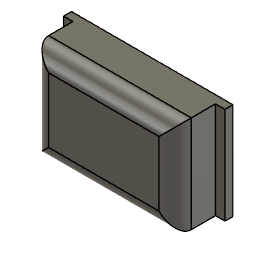
Side-Button (Autodesk Fusion 360 design; units mm, degrees)
Autodesk Fusion 360 part; units mm, degrees
sketch "Sketch1" plane through (0, 0, 0) normal (0, 0, 1) x (1, 0, 0)
  line L0 (-30, 20) -> (-12.335, 20)
  line L1 (-12.335, 20) -> (-12.335, 8)
  line L2 (-12.335, 8) -> (-30, 8)
  line L3 (-30, 8) -> (-30, 20)
  dimension "d1" = 17.665
  dimension "d2" = 12
  constraint horizontal L0
  constraint vertical L1
  constraint horizontal L2
  constraint vertical L3
  measures "d1" distance of L0.start L0.end
  measures "d2" distance of L0.start L2.end
extrude "Extrude1" add sketch "Sketch1" along normal blind 6
fillet "Fillet1" radius 2 4 edges at (-21.1675, 20, 6) (-12.335, 14, 6) (-30, 14, 6) (-21.1675, 8, 6)
sketch "Sketch2" plane through (0, 0, 0) normal (0, 0, -1) x (-1, 0, 0)
  line L0 (12.335, 8) -> (30, 8)
  line L1 (30, 8) -> (30, 20)
  line L2 (30, 20) -> (12.335, 20)
  line L3 (12.335, 20) -> (12.335, 8)
  line L4 (11.1675, 20) -> (31.1675, 20)
  line L5 (11.1675, 8) -> (31.1675, 8)
  line L6 (31.1675, 20) -> (31.1675, 8)
  line L7 (11.1675, 8) -> (11.1675, 20)
  point P0 (21.1675, 20)
  point P1 (21.1675, 8)
  dimension "d7" = 20
  constraint midpoint L4 P0
  constraint coincident L2 P0
  constraint parallel L2 L4
  constraint midpoint L5 P1
  constraint coincident L0 P1
  constraint perpendicular L1 L5
  constraint perpendicular L5 L6
  constraint perpendicular L4 L7
  measures "d7" distance of L4.start L4.end
extrude "Extrude2" add sketch "Sketch2" against normal blind 1 contours L3 L4 L5 L7 | L1 L4 L5 L6
